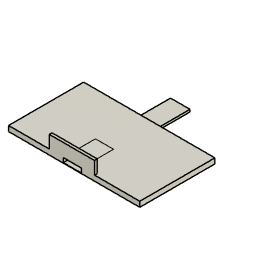
Phone Hollder v1 (Autodesk Fusion 360 design; units mm, degrees)
Autodesk Fusion 360 part; units mm, degrees
sketch "Sketch1" plane through (0, 0, 0) normal (0, 0, 1) x (1, 0, 0)
  line L0 (-25, 25) -> (-4, 25)
  line L1 (-4, 25) -> (-4, -11)
  line L2 (-4, -11) -> (-25, -11)
  line L3 (-25, -11) -> (-25, 25)
  dimension "d1" = 21
  dimension "d2" = 36
  constraint horizontal L0
  constraint vertical L1
  constraint horizontal L2
  constraint vertical L3
  measures "d1" distance of L0.start L0.end
  measures "d2" distance of L0.start L2.end
extrude "Extrude1" add sketch "Sketch1" along normal blind 5.8
shell "Shell1" thickness 0.5 removed faces 1 at (-18, -11, 3.8667)
sketch "Sketch2" plane through (0, 0, 5.8) normal (0, 0, 1) x (-1, 0, 0)
  line L0 (25, 11) -> (4, 11)
  line L1 (4, 11) -> (4, -25)
  line L2 (4, -25) -> (25, -25)
  line L3 (25, -25) -> (25, 11)
  line L4 (85, -72) -> (-60, -72)
  line L5 (-60, -72) -> (-60, 11)
  line L6 (-60, 11) -> (85, 11)
  line L7 (85, 11) -> (85, -72)
  line L8 (40, 11) -> (-10, 11)
  line L9 (-10, 11, 0) -> (-10, 11, 14)
  line L10 (-10, 11, 14) -> (40, 11, 14)
  line L11 (40, 11, 14) -> (40, 11, 0)
  dimension "d6" = 145
  dimension "d7" = 83
  dimension "d8" = 14
  constraint horizontal L4
  constraint vertical L5
  constraint horizontal L6
  constraint vertical L7
  constraint horizontal L8
  measures "d6" distance of L4.start L4.end
  measures "d7" distance of L4.start L6.end
extrude "Extrude2" add sketch "Sketch2" against normal blind 5.8 contours L1 L2 L3 L4 L5 L6 L7 L8
extrude "Extrude3" add sketch "Sketch2" against normal blind 3 contours L0 L6 L8 L9 L10 L11 in plane through (0, -11, 5.8) normal (0, -1, 0)
sketch "Sketch4" plane through (0, 0, 0) normal (0, 0, 1) x (1, 0, 0)
  line L0 (-3.5, 72) -> (-25, 72)
  line L1 (-25, 72) -> (-25, 108)
  line L2 (-25, 108) -> (-3.5, 108)
  line L3 (-3.5, 108) -> (-3.5, 72)
  dimension "d13" = 21.5
  dimension "d14" = 36
  constraint horizontal L0
  constraint vertical L1
  constraint horizontal L2
  constraint vertical L3
  measures "d13" distance of L0.start L0.end
  measures "d14" distance of L0.start L2.end
extrude "Extrude4" add sketch "Sketch4" along normal blind 2.5
